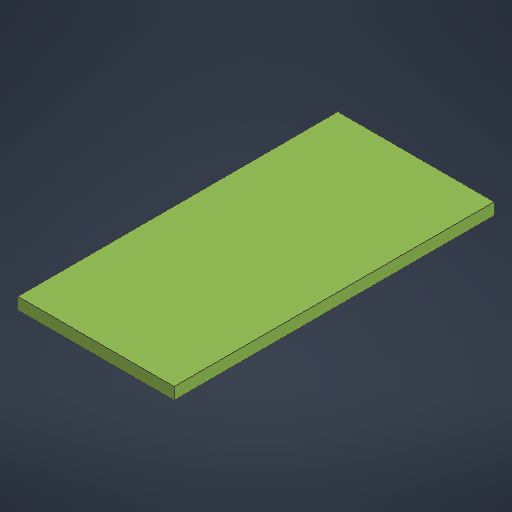
# Autodesk Inventor part: buck_converter
Saved by Autodesk Inventor 2026.2 (Build 302298010, 298A)
## iProperties
Created: 2026-07-05
Part Number: buck_converter
Material: Generic
Document SubType Name: Modeling
Designer: vicke
Density: 1 g/cm^3
Appearance: Default
Author: vicke
Autodesk Inventor part; units mm, degrees
ref_plane "YZ Plane" through (0, 0, 0) normal (1, 0, 0) x (0, 1, 0)
ref_plane "XZ Plane" through (0, 0, 0) normal (0, 1, 0) x (-1, 0, 0)
ref_plane "XY Plane" through (0, 0, 0) normal (0, 0, 1) x (1, 0, 0)
sketch "Sketch2" plane through (0, 0, 0) normal (0, 1, 0) x (-1, 0, 0)
  line L0 (0, 0) -> (21, 0)
  line L1 (21, 0) -> (21, -43)
  line L2 (21, -43) -> (0, -43)
  line L3 (0, -43) -> (0, 0)
  dimension "d0" = 43
  dimension "d1" = 21
  constraints: 8 end point, 2 parallel, 1 horizontal, 1 perpendicular
  measures "d0" distance between parallel lines of L0 L2
  measures "d1" distance between parallel lines of L3 L1
extrude "Extrusion1" add sketch "Sketch2" along normal blind 1.6
body "Solid1"
